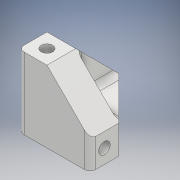
# Autodesk Inventor part: connector
Saved by Autodesk Inventor 2017 (Build 210142000, 142)
## iProperties
Created: 2019-02-08
Part Number: connector
Material: ABS Plastic
Document SubType Name: Modeling
Designer: felix
Density: 1.06 g/cm^3
Appearance: Smooth - White
Author: felix
Autodesk Inventor part; units mm, degrees
ref_plane "YZ Plane" through (0, 0, 0) normal (1, 0, 0) x (0, 1, 0)
ref_plane "XZ Plane" through (0, 0, 0) normal (0, 1, 0) x (-1, 0, 0)
ref_plane "XY Plane" through (0, 0, 0) normal (0, 0, 1) x (1, 0, 0)
sketch "Sketch1" plane through (0, 0, 0) normal (0, 0, 1) x (1, 0, 0)
  circle A0 centre (0, 0) radius 4
  line L0 (-10, -10) -> (10, -10)
  line L1 (10, -10) -> (10, 10)
  line L2 (10, 10) -> (-10, 10)
  line L3 (-10, 10) -> (-10, -10)
  line L4 (-10, -10) -> (10, 10) construction
  line L5 (10, -10) -> (-10, 10) construction
  dimension "d0" = 8
  dimension "d3" = 20
  dimension "d4" = 10
  dimension "d5" = 10
  constraints: 12 end point, 2 parallel, 2 perpendicular, 1 centre point, 1 coincident, 1 horizontal
  measures "d0" diameter of A0
  measures "d3" distance between parallel lines of L1 L3
  measures "d4" distance from line of point (0, 0) L1
  measures "d5" distance from line of point (0, 0) L2
extrude "Extrusion1" add sketch "Sketch1" along normal blind 30 and the other way blind 20
extrude "Extrusion2" add sketch "Sketch1" against normal up to surface (20 mm away) contours A0
sketch "Sketch2" plane through (-10, -10, 30) normal (-1, 0, 0) x (0, 0, 1)
  line L0 (-50, 20) -> (-50, 0) projected
  line L1 (-50, 20) -> (-30, 20)
  line L2 (-30, 20) -> (-30, 0)
  line L3 (-30, 0) -> (-50, 0)
  line L4 (-50, 0) -> (-50, 20)
  point P0 (-30, 10)
  constraints: 8 end point, 2 parallel, 1 horizontal, 1 perpendicular
extrude "Extrusion3" add sketch "Sketch2" along normal blind 30
sketch "Sketch3" plane through (-10, -10, 30) normal (0, -1, 0) x (1, 0, 0)
  line L0 (0, -30) -> (-30, -30) projected
  line L1 (0, -30) -> (20, -30)
  line L2 (20, -30) -> (20, -50)
  line L3 (20, -50) -> (0, -50)
  line L4 (0, -50) -> (0, -30)
  point P0 (10, -30)
  constraints: 8 end point, 2 parallel, 1 horizontal, 1 perpendicular
extrude "Extrusion4" add sketch "Sketch3" along normal blind 30
sketch "Sketch4" plane through (-40, -10, 30) normal (-1, 0, 0) x (0, 0, 1)
  circle A0 centre (-40, 10) radius 4
  point P0 (-30, 10)
  dimension "d16" = 8
  constraints: 1 centre point
  measures "d16" diameter of A0
extrude "Extrusion5" cut sketch "Sketch4" against normal blind 30
sketch "Sketch5" plane through (-10, -40, 30) normal (0, -1, 0) x (1, 0, 0)
  circle A0 centre (10, -40) radius 4
  point P0 (10, -30)
  dimension "d19" = 8
  constraints: 1 centre point
  measures "d19" diameter of A0
extrude "Extrusion6" cut sketch "Sketch5" against normal blind 30
sketch "Sketch6" plane through (0, 0, -20) normal (0, 0, -1) x (-1, 0, 0)
  line L0 (10, -10) -> (40, -10) projected
  line L1 (10, -10) -> (10, -40) projected
  line L2 (10, -40) -> (-10, -40) projected
  line L3 (40, -10) -> (10, -40)
  point P0 (0, 0)
  constraints: 2 end point
extrude "Extrusion7" add sketch "Sketch6" against normal blind 20
sketch "Sketch7" plane through (-10, 10, 30) normal (0, 1, 0) x (1, 0, 0)
  line L0 (-30, 30) -> (-30, 50) projected
  line L1 (0, 30) -> (-30, 30) projected
  line L2 (-30, 30) -> (0, 30)
  line L3 (0, 0) -> (20, 0) projected
  line L4 (0, 30) -> (0, 0)
  line L5 (0, 0) -> (-30, 30)
  point P0 (10, 30)
  constraints: 6 end point, 1 collinear, 1 perpendicular
extrude "Extrusion8" add sketch "Sketch7" against normal blind 20
sketch "Sketch8" plane through (10, -10, 30) normal (1, 0, 0) x (0, 0, -1)
  line L0 (30, 0) -> (0, 0) projected
  line L1 (30, 0) -> (30, -30) projected
  line L2 (0, 20) -> (0, 0) projected
  line L3 (0, 0) -> (30, -30)
  point P0 (30, 10)
  constraints: 2 end point
extrude "Extrusion9" add sketch "Sketch8" against normal blind 20
sketch "Sketch9" plane through (10, 10, 30) normal (0, 1, 0) x (1, 0, 0)
  line L0 (-50, 36) -> (-20, 36) projected
  line L1 (-14, 30) -> (-14, 0) projected
  circle A0 centre (-26.3015, 23.6985) radius 12.3015
  line L2 (-50, 30) -> (-20, 0) projected
  point P0 (-10, 30)
  constraints: 3 tangent, 1 centre point, 1 coincident
hole "Hole1" at (-16.3015, 10, 6.3015) direction (0, -1, 0) diameter 3.5 end through all
fillet "Fillet1" radius 4 3 edges at (-10, -25, 0) (-10, -10, 15) (-25, -10, 0)
fillet "Fillet2" radius 4 1 edges at (10, -15, -20)
fillet "Fillet3" radius 4 2 edges at (10, 0, 30) (-40, 0, -20)
move or copy body "Move Body1" bodies to move or copy 1 copy no rotation origin (0, 0, 0) rotation axis (-0.5773503, 0.5773503, -0.5773503) rotation angle 120 translate (30, 20, -10)
body "Solid1"
